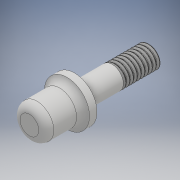
# Autodesk Inventor part: 零件1
Saved by Autodesk Inventor 2018.2 (Build 222227000, 227)
## iProperties
Created: 2017-12-27
Part Number: 零件1
Material: 常规
Document SubType Name: Modeling
Designer: Administrator
Density: 1 g/cm^3
Appearance: 默认
Author: Administrator
Autodesk Inventor part; units mm, degrees
ref_plane "YZ Plane" through (0, 0, 0) normal (1, 0, 0) x (0, 1, 0)
ref_plane "XZ Plane" through (0, 0, 0) normal (0, 1, 0) x (-1, 0, 0)
ref_plane "XY Plane" through (0, 0, 0) normal (0, 0, 1) x (1, 0, 0)
sketch "草图1" plane through (0, 0, 0) normal (0, 1, 0) x (-1, 0, 0)
  circle A0 centre (0, 0) radius 3
  circle A1 centre (0, 0) radius 6
  dimension "d0" = 6
  dimension "d10" = 12
  constraints: 2 centre point, 2 coincident
  measures "d0" diameter of A0
  measures "d10" diameter of A1
extrude "拉伸3" add sketch "草图1" against normal blind 2 contours A0 | A1
extrude "拉伸4" add sketch "草图1" along normal blind 20 contours A0
thread "螺纹6" size "M6x1" class "6g" standard "ANSI Metric M Profile" length 10
sketch "草图6" plane through (0, 20, 0) normal (1, 0, 0) x (0, 0, 1)
  line L0 (3, 0) -> (3, 10)
  line L1 (3, 10) -> (2.4587, 10)
  line L2 (2.4587, 10) -> (2.4587, 0)
  line L3 (2.4587, 0) -> (3, 0)
  line L4 (0, -4.4) -> (0, 26.4) projected
  constraints: 8 end point
revolve "旋转3" cut sketch "草图6" angle 360 about axis through (0, 20, 0) along (0, -1, 0)
sketch "草图7" plane through (0, 20, 0) normal (1, 0, 0) x (0, 0, 1)
  line L0 (3, 0) -> (3, 10)
  line L1 (3, 10) -> (2.4587, 10)
  line L2 (2.4587, 10) -> (2.4587, 0)
  line L3 (2.4587, 0) -> (3, 0)
  line L4 (0, -4.4) -> (0, 26.4) projected
  constraints: 8 end point
revolve "旋转4" add sketch "草图7" angle 360 about axis through (0, 20, 0) along (0, -1, 0) separate body
sketch "草图5" plane through (0, 20, 0) normal (-1, 0, 0) x (0, -1, 0)
  line L0 (-0.5, -2.2422) -> (-0.6611, -2.5212) construction
  line L1 (-0.5, -2.2422) -> (-0.3389, -2.5212) construction
  line L2 (-0.5, -2.2422) -> (-0.5, -2.4587) construction
  line L3 (-0.625, -2.4587) -> (-0.5528, -2.4587) construction
  line L4 (0, -3.1083) -> (0.0625, -3) construction
  line L5 (-1, -3.1083) -> (-1.0625, -3) construction
  line L6 (-1.0625, -3) -> (-1, -3) construction
  line L7 (-0.9375, -3) -> (-1, -3.1083) construction
  arc A0 (-0.5528, -2.4587) -> (-0.6611, -2.5212) centre (-0.5528, -2.5837) ccw
  arc A1 (-0.3389, -2.5212) -> (-0.4472, -2.4587) centre (-0.4472, -2.5837) ccw
  line L8 (0, -3.1083) -> (0, -3) construction
  line L9 (-1, -3.1083) -> (-1, -3) construction
  arc A2 (-0.0805, -2.9688) -> (-0.0264, -3) centre (-0.0264, -2.9375) ccw
  line L10 (-0.3389, -2.5212) -> (-0.0805, -2.9688)
  line L11 (-0.5528, -2.4587) -> (-0.4472, -2.4587)
  line L12 (-0.6611, -2.5212) -> (-0.9195, -2.9688)
  line L13 (-0.0264, -3) -> (0, -3) construction
  line L14 (0, -3) -> (0.0625, -3) construction
  arc A3 (-0.9736, -3) -> (-0.9195, -2.9688) centre (-0.9736, -2.9375) ccw
  line L15 (-0.9195, -2.9688) -> (-0.9375, -3) construction
  line L16 (-1, -3) -> (-0.9736, -3) construction
  line L17 (-0.9736, -3) -> (-0.0264, -3)
  line L18 (0, 0) -> (0.4413, 0)
  line L19 (0, 0) -> (0, 0.419)
  line L20 (0, -3.1083) -> (-0.0805, -2.9688) construction
  dimension "d53" = 0.2165
  dimension "d54" = 0.125
  dimension "d55" = 0.0625
  dimension "d56" = 0.1082
  dimension "d57" = 1
  dimension "草图5_MajorRadius" = 3
  dimension "d59" = 60
  dimension "草图5_ThreadOffset" = 0
  dimension "草图5_MinorRadius" = 2.4587
  constraints: 42 end point, 17 tangent, 8 point on circle, 6 parallel, 5 collinear, 4 centre point, 3 point on line, 3 vertical, 2 equal radius, 2 horizontal, 2 perpendicular, 1 equal length, 1 midpoint, 4 other
  measures "d53" distance from line of L0.start L3
  measures "d54" radius of A0
  measures "d55" radius of A2
  measures "d56" distance from line of L14 L4.start
  measures "d57" distance between parallel lines of L8 L9
  measures "草图5_MajorRadius" distance between parallel lines of L14 L18
  measures "d59" angle of L10 L12
  measures "草图5_ThreadOffset" distance between parallel lines of L19 L8
  measures "草图5_MinorRadius" distance between parallel lines of L18 L11
coil "螺旋扫掠3" sketch "草图5" operation cut axis through (0, 20, 0) along (0, -1, 0) pitch 1.001 turns 11.988012 hand right bodies 2
sketch "草图8" plane through (0, -2, 0) normal (0, -1, 0) x (1, 0, 0)
  circle A0 centre (0, 0) radius 6 projected
  circle A1 centre (0, 0) radius 4.5
  dimension "d75" = 9
  constraints: 1 centre point, 1 coincident
  measures "d75" diameter of A1
extrude "拉伸5" add sketch "草图8" along normal blind 10 contours A1 bodies 1
fillet "圆角1" radius 2 1 edges at (-4.5, -2, 0)
fillet "圆角2" radius 2 1 edges at (-4.5, -12, 0)
equation "\"d53\" = 0.216506 * 草图5_Pitch"
equation "\"d54\" = d62"
equation "\"d55\" = 0.0625 * 草图5_Pitch"
equation "\"d56\" = 0.108253 * 草图5_Pitch"
equation "\"d57\" = 草图5_Pitch"
equation "\"d59\" = d64"
equation "\"d38\" = 0.125 * 草图2_Pitch"
equation "\"草图2_Pitch\" = 1"
equation "\"d40\" = 60deg"
equation "\"d62\" = 0.125 * 草图5_Pitch"
equation "\"草图5_Pitch\" = 1"
equation "\"d64\" = 60deg"
